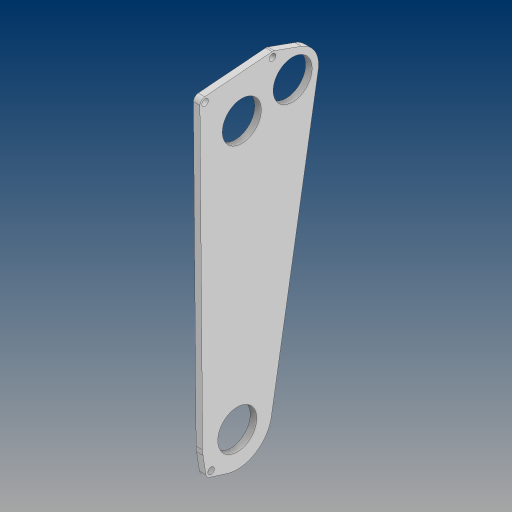
# Autodesk Inventor part: INTK_001_PulleyCover2
Saved by Autodesk Inventor 2024.3 (Build 283343000, 343)
## iProperties
Created: 2024-08-03
Part Number: INTK_001_PulleyCover2
Material: Generic
Document SubType Name: Modeling
Designer: Kenji
Density: 1 g/cm^3
Appearance: Default
Author: Kenji
Autodesk Inventor part; units mm, degrees
ref_plane "YZ Plane" through (0, 0, 0) normal (1, 0, 0) x (0, 1, 0)
ref_plane "XZ Plane" through (0, 0, 0) normal (0, 1, 0) x (-1, 0, 0)
ref_plane "XY Plane" through (0, 0, 0) normal (0, 0, 1) x (1, 0, 0)
sketch "Sketch1" plane through (0, 0, 0) normal (1, 0, 0) x (0, 1, 0)
  circle A0 centre (0, 0) radius 25.4 construction
  line L0 (0, 0) -> (0, -40.64) construction
  line L1 (0, -40.64) -> (202.057, -40.64) construction
  circle A1 centre (202.057, -40.64) radius 19.05 construction
  line L2 (202.057, -40.64) -> (194.4116, -40.64) construction
  line L3 (194.4116, -40.64) -> (194.4116, -3.3274) construction
  circle A2 centre (194.4116, -3.3274) radius 30.48 construction
  line L4 (16.6237, -19.2045) -> (-16.6237, 19.2045) construction
  circle A3 centre (-16.6237, 19.2045) radius 2.3876
  circle A4 centre (-16.6237, 19.2045) radius 3.81 construction
  line L5 (215.2378, 18.9279) -> (216.9733, 20.7826) construction
  line L6 (218.4988, -22.0046) -> (220.5061, -23.561) construction
  line L7 (194.4116, -3.3274) -> (194.4116, 27.1526) construction
  circle A5 centre (223.5169, -25.8957) radius 2.3876
  circle A6 centre (219.5766, 23.5645) radius 2.3876
  circle A7 centre (219.5766, 23.5645) radius 3.81 construction
  circle A8 centre (223.5169, -25.8957) radius 3.81 construction
  line L8 (223.3745, 23.8671) -> (227.3149, -25.5931)
  line L9 (227.1043, -27.1789) -> (219.9939, -47.0563)
  line L10 (198.8779, -59.4229) -> (-4.2389, -25.0438)
  arc A9 (227.1043, -27.1789) -> (227.3149, -25.5931) centre (223.5169, -25.8957) ccw
  arc A10 (198.8779, -59.4229) -> (219.9939, -47.0563) centre (202.057, -40.64) ccw
  line L11 (219.5423, 27.3743) -> (-0.2283, 25.399)
  line L12 (-4.0136, 25.0809) -> (-17.2257, 22.9666)
  line L13 (-20.2607, 20.3395) -> (-24.2467, 7.5667)
  arc A11 (-0.2283, 25.399) -> (-4.0136, 25.0809) centre (0, 0) ccw
  arc A12 (-17.2257, 22.9666) -> (-20.2607, 20.3395) centre (-16.6237, 19.2045) ccw
  arc A13 (-24.2467, 7.5667) -> (-4.2389, -25.0438) centre (0, 0) ccw
  arc A14 (223.3745, 23.8671) -> (219.5423, 27.3743) centre (219.5766, 23.5645) ccw
  circle A15 centre (194.4116, -3.3274) radius 14.2875
  circle A16 centre (202.057, -40.64) radius 14.2875
  circle A17 centre (0, 0) radius 14.2875
  dimension "d0" = 50.8
  dimension "d1" = 40.64
  dimension "d2" = 202.057
  dimension "d3" = 38.1
  dimension "d4" = 7.6454
  dimension "d5" = 37.3126
  dimension "d6" = 60.96
  dimension "d7" = 40.88
  dimension "d8" = 4.7752
  dimension "d9" = 7.62
  dimension "d10" = 2.54
  dimension "d11" = 2.54
  dimension "d12" = 43.1
  dimension "d13" = 127.79
  dimension "d14" = 4.7752
  dimension "d15" = 4.7752
  dimension "d16" = 7.62
  dimension "d17" = 7.62
  dimension "d18" = 28.575
  dimension "d19" = 28.575
  dimension "d20" = 28.575
  constraints: 31 point on circle, 28 end point, 18 centre point, 13 tangent, 10 coincident, 6 concentric, 5 point on line, 1 collinear, 1 horizontal, 1 midpoint, 1 perpendicular, 1 vertical
  measures "d0" diameter of A0
  measures "d1" distance of L0.start L0.end
  measures "d2" distance of L0.end L1.end
  measures "d3" diameter of A1
  measures "d4" distance of L2.start L2.end
  measures "d5" distance of L2.end L3.end
  measures "d6" diameter of A2
  measures "d7" angle of L4 L0
  measures "d8" diameter of A3
  measures "d9" diameter of A4
  measures "d10" distance of L5.start L5.end
  measures "d11" distance of L6.start L6.end
  measures "d12" angle of L7 L5
  measures "d13" angle of L6 L7
  measures "d14" diameter of A5
  measures "d15" diameter of A6
  measures "d16" diameter of A7
  measures "d17" diameter of A8
  measures "d18" diameter of A15
  measures "d19" diameter of A16
  measures "d20" diameter of A17
extrude "Extrusion1" add sketch "Sketch1" along normal blind 4.7625
body "Solid1"
